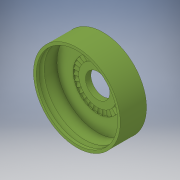
# Autodesk Inventor part: wheel hub
Saved by Autodesk Inventor 2018 (Build 220112000, 112)
## iProperties
Created: 2017-11-23
Part Number: wheel hub
Material: ABS Plastic
Document SubType Name: Modeling
Designer: prakh
Density: 1.06 g/cm^3
Appearance: Olive Green
Author: prakh
Autodesk Inventor part; units mm, degrees
ref_plane "YZ Plane" through (0, 0, 0) normal (1, 0, 0) x (0, 1, 0)
ref_plane "XZ Plane" through (0, 0, 0) normal (0, 1, 0) x (-1, 0, 0)
ref_plane "XY Plane" through (0, 0, 0) normal (0, 0, 1) x (1, 0, 0)
sketch "Sketch1" plane through (0, 0, 0) normal (0, 0, 1) x (1, 0, 0)
  circle A0 centre (0, 0) radius 50.7746
  line L0 (2.7496, 4.7625) -> (5.4993, 0)
  line L1 (5.4993, 0) -> (2.7496, -4.7625)
  line L2 (2.7496, -4.7625) -> (-2.7496, -4.7625)
  line L3 (-2.7496, -4.7625) -> (-5.4993, 0)
  line L4 (-5.4993, 0) -> (-2.7496, 4.7625)
  line L5 (-2.7496, 4.7625) -> (2.7496, 4.7625)
  circle A1 centre (0, 0) radius 14.2875
  dimension "d0" = 101.5492
  dimension "d3" = 9.525
  dimension "d22" = 28.575
  constraints: 12 end point, 3 coincident, 2 centre point, 13 other
  measures "d0" diameter of A0
  measures "d3" distance between parallel lines of L5 L2
  measures "d22" diameter of A1
extrude "Extrusion1" add sketch "Sketch1" along normal blind 3.175 contours A0
sketch "Sketch3" plane through (0, 0, 3.175) normal (0, 0, 1) x (1, 0, 0)
  circle A0 centre (0, 0) radius 22.225
  circle A1 centre (0, 0) radius 28.575
  dimension "d4" = 44.45
  dimension "d6" = 6.35
  constraints: 2 centre point, 2 coincident
  measures "d4" diameter of A0
  measures "d6" radial gap between concentric circles of A1 A0
extrude "Extrusion2" add sketch "Sketch3" along normal blind 3.175
sketch "Sketch4" plane through (0, 0, 0) normal (1, 0, 0) x (0, 1, 0)
  line L0 (28.575, 6.35) -> (-28.575, 6.35) projected
  arc A0 (-2.7496, 6.35) -> (2.7496, 6.35) centre (0, 7.9375) ccw
  point P0 (0, 0)
  dimension "d9" = 3.175
  dimension "d10" = 1.5875
  constraints: 2 point on circle, 2 point on line, 1 centre point, 1 vertical alignment
  measures "d9" radius of A0
  measures "d10" distance from line of A0.centre L0
extrude "Extrusion3" cut sketch "Sketch4" along normal blind 31.75
pattern_circular "Circular Pattern1" count 30 over 360 about axis through (0, 0, -10) along (0, 0, 1) of "Extrusion3"
sketch "Sketch5" plane through (0, 0, 3.175) normal (0, 0, 1) x (1, 0, 0)
  circle A0 centre (0, 0) radius 22.225
  circle A1 centre (0, 0) radius 19.05
  circle A2 centre (0, 0) radius 28.575
  circle A3 centre (0, 0) radius 31.75
  circle A4 centre (0, 0) radius 50.7746 projected
  circle A5 centre (0, 0) radius 22.225 projected
  circle A6 centre (0, 0) radius 14.2875 projected
  dimension "d16" = 3.175
  dimension "d17" = 44.45
  dimension "d18" = 57.15
  dimension "d19" = 3.175
  constraints: 4 centre point, 4 coincident
  measures "d16" radial gap between concentric circles of A1 A0
  measures "d17" diameter of A0
  measures "d18" diameter of A2
  measures "d19" radial gap between concentric circles of A2 A3
extrude "Extrusion4" add sketch "Sketch5" along normal up to surface (3.175 mm away) contours A0 | A1 | A3 | A4
sketch "Sketch6" plane through (0, 0, 0) normal (1, 0, 0) x (0, 1, 0)
  line L0 (-50.7746, 6.35) -> (50.7746, 6.35) projected
  line L1 (-50.7746, 0) -> (50.7746, 0) projected
  line L2 (-50.7746, 6.35) -> (-47.625, 6.35)
  line L3 (-47.625, 30.6324) -> (-50.7746, 30.6324)
  line L4 (-50.7746, 30.6324) -> (-50.7746, 6.35)
  arc A0 (-47.625, 27.252) -> (-47.625, 21.3128) centre (-45.9105, 24.2824) ccw
  line L5 (-47.625, 6.35) -> (-47.625, 21.3128)
  line L6 (-47.625, 27.252) -> (-47.625, 30.6324)
  line L7 (0, -6.1265) -> (0, 36.7589) projected
  point P0 (0, 0)
  dimension "d23" = 3.429
  dimension "d24" = 17.9324
  dimension "d27" = 24.2824
  dimension "d30" = 1.7145
  dimension "d31" = 47.625
  constraints: 10 end point, 3 parallel, 2 perpendicular, 2 point on circle, 1 centre point, 1 collinear, 1 horizontal
  measures "d23" radius of A0
  measures "d24" distance from line of A0.centre L0
  measures "d27" distance of L3.end L0.start
  measures "d30" distance centre to line of A0 L5
  measures "d31" distance from line of L5 point (0, 0)
revolve "Revolution1" add sketch "Sketch6" angle 360 about axis through (0, 0, -10) along (0, 0, 1)
equation "\"d16\" = d19"
body "Solid1"
